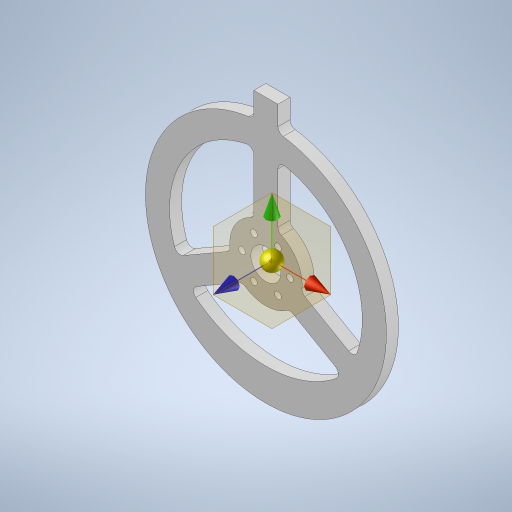
# Autodesk Inventor part: Emma Blade
Saved by Autodesk Inventor 2023.2 (Build 272271000, 271)
## iProperties
Created: 2023-03-02
Part Number: Emma Blade
Material: Generic
Document SubType Name: Modeling
Designer: Nathan Cai
Mass: 45.1572 g
Surface Area: 210.425 cm^2
Volume: 45.1572 cm^3
Density: 1 g/cm^3
Appearance: Default
Author: Nathan Cai
Autodesk Inventor part; units mm, degrees
ref_plane "YZ Plane" through (0, 0, 0) normal (1, 0, 0) x (0, 1, 0)
ref_plane "XZ Plane" through (0, 0, 0) normal (0, 1, 0) x (-1, 0, 0)
ref_plane "XY Plane" through (0, 0, 0) normal (0, 0, 1) x (1, 0, 0)
sketch "Sketch1" plane through (0, 0, 0) normal (0, 0, 1) x (1, 0, 0)
  circle A0 centre (0, 0) radius 63.5
  line L0 (0, 0) -> (0, 63.5) construction
  line L1 (-6.35, 76.2) -> (6.35, 76.2)
  line L2 (6.35, 76.2) -> (6.35, 0)
  line L3 (6.35, 0) -> (-6.35, 0) construction
  line L4 (-6.35, 0) -> (-6.35, 76.2)
  line L5 (-6.35, 76.2) -> (6.35, 0) construction
  line L6 (6.35, 76.2) -> (-6.35, 0) construction
  circle A1 centre (0, 0) radius 50.8
  circle A2 centre (0, 0) radius 19.05
  line L7 (-69.1661, -32.6007) -> (-3.175, 5.4993)
  line L8 (3.175, -5.4993) -> (-62.8161, -43.5993)
  line L9 (62.8161, -43.5993) -> (-3.175, -5.4993)
  line L10 (3.175, 5.4993) -> (69.1661, -32.6007)
  circle A3 centre (0, 0) radius 12.7 construction
  circle A4 centre (6.35, 10.9985) radius 1.7526
  line L11 (0, 0) -> (6.35, 10.9985) construction
  circle A5 centre (-6.35, 10.9985) radius 1.7526
  circle A6 centre (-12.7, 0) radius 1.7526
  circle A7 centre (-6.35, -10.9985) radius 1.7526
  circle A8 centre (6.35, -10.9985) radius 1.7526
  circle A9 centre (12.7, 0) radius 1.7526
  circle A10 centre (0, 0) radius 7.9375
  circle A11 centre (0, 57.15) radius 3.175
  arc A12 (-40.474, -30.7) -> (40.474, -30.7) centre (0, 13.0686) ccw
  point P0 (0, 38.1)
  point P1 (-6.35, 50.4016)
  point P2 (-6.35, 17.9605)
  point P3 (-18.7293, -3.481)
  point P4 (-46.824, -19.7015)
  point P5 (-6.35, 63.1817)
  point P6 (6.35, 63.1817)
  point P7 (-12.3793, -14.4795)
  point P8 (12.3793, -14.4795)
  point P9 (40.474, -30.7)
  point P10 (6.35, 50.4016)
  point P11 (46.824, -19.7015)
  point P12 (18.7293, -3.481)
  point P13 (6.35, 17.9605)
  point P14 (0, -46.5455)
  dimension "d0" = 127
  dimension "d9" = 25.4
  dimension "d1" = 76.2
  dimension "d2" = 12.7
  dimension "d3" = 12.7
  dimension "d4" = 38.1
  dimension "d7" = 360
  dimension "d10" = 3.5052
  dimension "d11" = 30
  dimension "d14" = 360
  dimension "d16" = 15.875
  dimension "d17" = 6.35
  dimension "d18" = 57.15
  dimension "d22" = 46.5455
  constraints: 24 end point, 11 centre point, 5 coincident, 5 point on circle, 4 midpoint, 4 point on line, 2 parallel, 1 horizontal, 1 perpendicular, 1 vertical, 38 other
  measures "d1" distance from line of point (0, 0) L1
  measures "d2" distance between parallel lines of L4 L2
  measures "d4" diameter of A2
  measures "d10" diameter of A4
  measures "d11" angle of L0 L11
  measures "d16" diameter of A10
  measures "d17" diameter of A11
  measures "d18" distance of A10.centre A11.centre
  measures "d22" distance of point (0, 0) point (0, -46.546)
extrude "Extrusion1" add sketch "Sketch1" along normal blind 6.35 contours A0 L10 A1 L2 | L2 A1 L4 A0 | A0 L4 L1 L2 | A0 L9 A1 L10 | L4 A1 L7 A0 | L2 A2 L4 A1 | A0 L8 A1 L9 | A1 L9 A2 L10 | L7 A1 L8 A0 | A2 L10 A9 A10 L2 A4 | L2 A4 A10 L4 A5 A2 | A1 A12 | A2 L9 A8 A10 L10 A9 | L7 A2 L8 A1 | L4 A5 A10 L7 A6 A2 | A2 L8 A7 A10 L9 A8 | L7 A6 A10 L8 A7 A2 | A11
fillet "Fillet1" radius 3.175 14 edges at (6.35, 50.4016, 3.175) (6.35, 17.9605, 3.175) (18.7293, -3.481, 3.175) (46.824, -19.7015, 3.175) (12.3793, -14.4795, 3.175) (-12.3793, -14.4795, 3.175) (-18.7293, -3.481, 3.175) (-6.35, 17.9605, 3.175) (-46.824, -19.7015, 3.175) (-6.35, 50.4016, 3.175) (-6.35, 63.1817, 3.175) (6.35, 63.1817, 3.175) (40.474, -30.7, 3.175) (-40.474, -30.7, 3.175)
body "Solid1"
